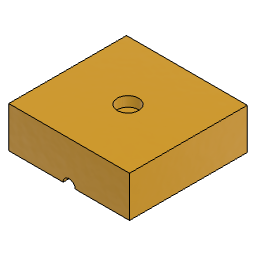
Tool change - one magnet (Autodesk Fusion 360 design; units mm, degrees)
Autodesk Fusion 360 part; units mm, degrees
note: some values were not read from the file. Chosen so that the rebuilt part matches the saved one: which face or edge a step refers to.
sketch "Sketch1" plane through (0, 0, 0) normal (0, 0, 1) x (1, 0, 0)
  line L0 (0, 1.3314) -> (42, 1.3314)
  line L1 (42, 1.3314) -> (42, 43.3314)
  line L2 (42, 43.3314) -> (0, 43.3314)
  line L3 (0, 43.3314) -> (0, 1.3314)
  dimension "d1" = 42
  dimension "d2" = 42
  constraint horizontal L0
  constraint vertical L1
  constraint horizontal L2
  constraint vertical L3
  measures "d1" distance of L0.start L2.end
  measures "d2" distance of L0.start L0.end
extrude "Extrude1" add sketch "Sketch1" along normal blind 7
sketch "Sketch2" plane through (0, 0, 7) normal (0, 0, 1) x (-1, 0, 0)
  line L0 (0, -43.3314) -> (0, -1.3314)
  line L1 (0, -1.3314) -> (-42, -1.3314)
  line L2 (-42, -1.3314) -> (-42, -43.3314)
  line L3 (-42, -43.3314) -> (0, -43.3314)
  circle A0 centre (-13, -22.3314) radius 3.55
  circle A1 centre (-29, -23.2838) radius 3.55
  dimension "d5" = 7.1
  dimension "d6" = 7.1
  dimension "d7" = 13
  dimension "d8" = 13
  dimension "d9" = 21
  measures "d5" diameter of A0
  measures "d6" diameter of A1
  measures "d7" distance of L0 A0.centre
  measures "d8" distance of L2 A1.centre
  measures "d9" distance of L1 A0.centre
sketch "Sketch4" plane through (0, 0, 7) normal (0, 0, 1) x (-1, 0, 0)
  line L0 (0, -43.3314) -> (0, -1.3314)
  line L1 (0, -1.3314) -> (-42, -1.3314)
  line L2 (-42, -1.3314) -> (-42, -43.3314)
  line L3 (-42, -43.3314) -> (0, -43.3314)
  circle A0 centre (-21, -22.3314) radius 3.55
  dimension "d12" = 7.1
  dimension "d13" = 21
  dimension "d14" = 21
  measures "d12" diameter of A0
  measures "d13" distance of L3 A0.centre
  measures "d14" distance of L0 A0.centre
extrude "Extrude3" cut sketch "Sketch4" against normal blind 3.3 contours A0
sketch "Sketch5" plane through (0, 0, 0) normal (0, 0, -1) x (1, 0, 0)
  line L0 (0, -1.3314) -> (0, -43.3314)
  line L1 (0, -43.3314) -> (42, -43.3314)
  line L2 (42, -43.3314) -> (42, -1.3314)
  line L3 (42, -1.3314) -> (0, -1.3314)
sketch "Sketch6" plane through (0, 0, 0) normal (0, 0, -1) x (1, 0, 0)
sketch "Sketch7" plane through (0, 0, 0) normal (0, 0, -1) x (1, 0, 0)
  line L0 (5.5, -6.1414) -> (36.5, -6.1414)
  line L1 (36.5, -6.1414) -> (36.5, -38.5214)
  line L2 (36.5, -38.5214) -> (5.5, -38.5214)
  line L3 (5.5, -38.5214) -> (5.5, -6.1414)
  line L4 (0, -1.3314) -> (0, -43.3314)
  line L5 (0, -43.3314) -> (42, -43.3314)
  line L6 (19, -6.1414) -> (23, -6.1414)
  line L7 (23, -6.1414) -> (23, -1)
  line L8 (23, -1) -> (19, -1)
  line L9 (19, -1) -> (19, -6.1414)
  line L10 (15.15, -38.5214) -> (26.85, -38.5214)
  line L11 (26.85, -38.5214) -> (26.85, -44)
  line L12 (26.85, -44) -> (15.15, -44)
  line L13 (15.15, -44) -> (15.15, -38.5214)
  line L14 (0, -1.3314) -> (42, -1.3314)
  line L15 (42, -1.3314) -> (42, -43.3314)
  line L16 (42, -43.3314) -> (0, -43.3314)
  line L17 (0, -43.3314) -> (0, -1.3314)
  dimension "d17" = 31
  dimension "d18" = 32.38
  dimension "d19" = 5.5
  dimension "d20" = 4.81
  dimension "d21" = 4
  dimension "d22" = 13.5
  dimension "d23" = 11.7
  dimension "d24" = 9.65
  constraint horizontal L0
  constraint vertical L1
  constraint horizontal L2
  constraint vertical L3
  constraint horizontal L6
  constraint vertical L7
  constraint horizontal L8
  constraint vertical L9
  constraint coincident L0 L6.start
  constraint horizontal L10
  constraint vertical L11
  constraint horizontal L12
  constraint vertical L13
  constraint coincident L2 L10.start
  constraint horizontal L14
  constraint vertical L15
  constraint horizontal L16
  constraint vertical L17
  constraint coincident L5.end L15.end
  constraint coincident L4.start L14.start
  measures "d17" distance of L0.start L0.end
  measures "d18" distance of L0.end L1.end
  measures "d19" distance of L3 L4
  measures "d20" distance of L2 L5
  measures "d21" distance of L7.end L8.end
  measures "d22" distance of L3 L9
  measures "d23" distance of L11.end L12.end
  measures "d24" distance of L3 L13
extrude "Extrude4" add sketch "Sketch7" along normal blind 6.55 contours L0 L2 L3 L4 L5 L9 L13 L14 L16 L17 | L0 L1 L2 L5 L7 L11 L14 L15 L16
sketch "Sketch8" plane through (0, 0, -6.55) normal (0, 0, -1) x (1, 0, 0)
  line L0 (15.15, -43.3314) -> (15.15, -38.5214)
  line L1 (15.15, -38.5214) -> (5.5, -38.5214)
  line L2 (5.5, -38.5214) -> (5.5, -6.1414)
  line L3 (5.5, -6.1414) -> (19, -6.1414)
  line L4 (19, -6.1414) -> (19, -1.3314)
  line L5 (19, -1.3314) -> (0, -1.3314)
  line L6 (0, -1.3314) -> (0, -43.3314)
  line L7 (0, -43.3314) -> (15.15, -43.3314)
sketch "Sketch9" plane through (0, 6.1414, 0) normal (0, 1, 0) x (-1, 0, 0)
  line L0 (-23, 0) -> (-36.5, 0)
  line L1 (-36.5, 0) -> (-36.5, -6.55)
  line L2 (-36.5, -6.55) -> (-23, -6.55)
  line L3 (-23, -6.55) -> (-23, 0)
sketch "Sketch10" plane through (0, 6.1414, 0) normal (0, 1, 0) x (-1, 0, 0)
  line L0 (-18.9881, 0) -> (-22.9881, 0)
  line L1 (-22.9881, 0) -> (-22.9881, -6.55)
  line L2 (-22.9881, -6.55) -> (-18.9881, -6.55)
  line L3 (-18.9881, -6.55) -> (-18.9881, 0)
  circle A0 centre (-20.9881, -6.55) radius 2
  dimension "d27" = 6.55
  dimension "d28" = 4
  dimension "d29" = 4
  constraint horizontal L0
  constraint vertical L1
  constraint horizontal L2
  constraint vertical L3
  constraint midpoint L2 A0.centre
  measures "d27" distance of L0.start L2.end
  measures "d28" distance of L1.end L2.end
  measures "d29" diameter of A0
sketch "Sketch11" plane through (0, 0, -6.55) normal (0, 0, -1) x (1, 0, 0)
  line L0 (23, -6.1414) -> (36.5, -6.1414)
  line L1 (36.5, -6.1414) -> (36.5, -38.5214)
  line L2 (36.5, -38.5214) -> (26.85, -38.5214)
  line L3 (26.85, -38.5214) -> (26.85, -43.3314)
  line L4 (26.85, -43.3314) -> (42, -43.3314)
  line L5 (42, -43.3314) -> (42, -1.3314)
  line L6 (42, -1.3314) -> (23, -1.3314)
  line L7 (23, -1.3314) -> (23, -6.1414)
sketch "Sketch12" plane through (0, 0, -6.55) normal (0, 0, -1) x (1, 0, 0)
extrude "Extrude9" add sketch "Sketch11" sketch "Sketch8" along normal blind 2 of sketch 2
sketch "Sketch22" plane through (0, 43.3314, 0) normal (0, 1, 0) x (-1, 0, 0)
  line L0 (-26.85, 0) -> (-15.15, 0)
  line L1 (-15.15, 0) -> (-15.15, -8.55)
  line L2 (-15.15, -8.55) -> (0, -8.55)
  line L3 (0, -8.55) -> (0, 7)
  line L4 (0, 7) -> (-42, 7)
  line L5 (-42, 7) -> (-42, -8.55)
  line L6 (-42, -8.55) -> (-26.85, -8.55)
  line L7 (-26.85, -8.55) -> (-26.85, 0)
  circle A0 centre (-21, -8) radius 5.85
  dimension "d42" = 11.7
  measures "d42" diameter of A0
sketch "Sketch23" plane through (0, 6.1414, 0) normal (0, 1, 0) x (-1, 0, 0)
sketch "Sketch24" plane through (0, 0, -8.55) normal (0, 0, -1) x (1, 0, 0)
  line L0 (23, -1.3314) -> (23, -6.1414)
  line L1 (23, -6.1414) -> (36.5, -6.1414)
  line L2 (36.5, -6.1414) -> (36.5, -38.5214)
  line L3 (36.5, -38.5214) -> (26.85, -38.5214)
  line L4 (26.85, -38.5214) -> (26.85, -43.3314)
  line L5 (26.85, -43.3314) -> (42, -43.3314)
  line L6 (42, -43.3314) -> (42, -1.3314)
  line L7 (42, -1.3314) -> (23, -1.3314)
sketch "Sketch25" plane through (0, 43.3314, 0) normal (0, 1, 0) x (-1, 0, 0)
extrude "Extrude10" add sketch "Sketch22" against normal blind 4.81 contours L0 L1 L7 A0
sketch "Sketch26" plane through (0, 6.1414, 0) normal (0, 1, 0) x (-1, 0, 0)
sketch "Sketch27" plane through (0, 1.3314, 0) normal (0, -1, 0) x (1, 0, 0)
  line L0 (19, 0) -> (23, 0)
  line L1 (23, 0) -> (23, -8.55)
  line L2 (23, -8.55) -> (42, -8.55)
  line L3 (42, -8.55) -> (42, 7)
  line L4 (42, 7) -> (0, 7)
  line L5 (0, 7) -> (0, -8.55)
  line L6 (0, -8.55) -> (19, -8.55)
  line L7 (19, -8.55) -> (19, 0)
  line L8 (23, -8.55) -> (19, -8.55)
  line L9 (23, -8.55) -> (23, 0)
  line L10 (19, -8.55) -> (19, 0)
  line L11 (23, 0) -> (19, 0)
  circle A0 centre (21, -8.55) radius 2
  dimension "d45" = 4
  constraint coincident L1.end L2.start
  constraint coincident L6.end L7.start
  constraint coincident L0.end L1.start
  constraint coincident L0.start L7.end
  constraint midpoint L8 A0.centre
  measures "d45" diameter of A0
extrude "Extrude11" add sketch "Sketch27" against normal blind 4.81 contours L0 L1 L7 L9 L10 L11 A0
sketch "Sketch28" plane through (36.5, 0, 0) normal (-1, 0, 0) x (0, -1, 0)
  line L0 (-6.1414, 0) -> (-38.5214, 0)
  line L1 (-38.5214, 0) -> (-38.5214, -8.55)
  line L2 (-38.5214, -8.55) -> (-6.1414, -8.55)
  line L3 (-6.1414, -8.55) -> (-6.1414, 0)
extrude "Extrude12" cut 1 faces at (0, 29.3314, -3.3667) along direction (1, 0, 0) blind 2
extrude "Extrude13" cut 1 faces at (42, 29.3314, 1.8167) along direction (-1, 0, 0) blind 2
extrude "Extrude14" cut 1 faces at (20.9502, 1.3314, 2.4815) along direction (0, 1, 0) blind 1.5
extrude "Extrude15" cut 1 faces at (6.5764, 43.3314, -2.3373) along direction (0, -1, 0) blind 1.5
sketch "Sketch29" plane through (0, 0, -8.55) normal (0, 0, -1) x (1, 0, 0)
  line L0 (2, -41.8314) -> (15.15, -41.8314)
  line L1 (15.15, -41.8314) -> (15.15, -38.5214)
  line L2 (15.15, -38.5214) -> (5.5, -38.5214)
  line L3 (5.5, -38.5214) -> (5.5, -6.1414)
  line L4 (5.5, -6.1414) -> (19, -6.1414)
  line L5 (19, -6.1414) -> (19, -2.8314)
  line L6 (19, -2.8314) -> (2, -2.8314)
  line L7 (2, -2.8314) -> (2, -41.8314)
extrude "Extrude16" add 1 faces at (20.9502, 2.8314, 2.4815) along direction (0, -1, 0) blind 0.5
extrude "Extrude17" add 1 faces at (6.5764, 41.8314, -2.3373) along direction (0, 1, 0) blind 0.5
extrude "Extrude18" add 1 faces at (40, 15.6647, 1.8167) along direction (1, 0, 0) blind 0.5
extrude "Extrude19" add 1 faces at (2, 15.6647, 1.8167) along direction (-1, 0, 0) blind 0.5
extrude "Extrude20" add 1 faces at (1.5, 15.6647, 1.8167) along direction (-1, 0, 0) blind 1
extrude "Extrude21" add 1 faces at (40.5, 15.6647, 1.8167) along direction (1, 0, 0) blind 1
sketch "Sketch30" plane through (0, 0, -8.55) normal (0, 0, -1) x (1, 0, 0)
  line L0 (41.5, -2.3314) -> (23, -2.3314)
  line L1 (23, -2.3314) -> (23, -6.1414)
  line L2 (23, -6.1414) -> (36.5, -6.1414)
  line L3 (36.5, -6.1414) -> (36.5, -38.5214)
  line L4 (36.5, -38.5214) -> (26.85, -38.5214)
  line L5 (26.85, -38.5214) -> (26.85, -42.3314)
  line L6 (26.85, -42.3314) -> (41.5, -42.3314)
  line L7 (41.5, -42.3314) -> (41.5, -2.3314)
extrude "Extrude22" cut 1 faces at (5.5764, 42.3314, -2.3373) along direction (0, -1, 0) blind 0.5
extrude "Extrude23" cut 1 faces at (21.0498, 2.3314, 2.4815) along direction (0, 1, 0) blind 0.5
extrude "Extrude24" cut 1 faces at (0.5, 15.8314, 1.8167) along direction (1, 0, 0) blind 0.5
extrude "Extrude25" cut 1 faces at (41.5, 15.8314, 1.8167) along direction (-1, 0, 0) blind 0.5
sketch "Sketch31" plane through (0, 0, -8.55) normal (0, 0, -1) x (1, 0, 0)
  line L0 (1, -2.8314) -> (1, -41.8314)
  line L1 (1, -41.8314) -> (15.15, -41.8314)
  line L2 (15.15, -41.8314) -> (15.15, -38.5214)
  line L3 (15.15, -38.5214) -> (5.5, -38.5214)
  line L4 (5.5, -38.5214) -> (5.5, -6.1414)
  line L5 (5.5, -6.1414) -> (19, -6.1414)
  line L6 (19, -6.1414) -> (19, -2.8314)
  line L7 (19, -2.8314) -> (1, -2.8314)
sketch "Sketch32" plane through (0, 0, -8.55) normal (0, 0, -1) x (1, 0, 0)
  line L0 (1, -2.8314) -> (1, -41.8314)
  line L1 (1, -41.8314) -> (15.15, -41.8314)
  line L2 (15.15, -41.8314) -> (15.15, -38.5214)
  line L3 (15.15, -38.5214) -> (5.5, -38.5214)
  line L4 (5.5, -38.5214) -> (5.5, -6.1414)
  line L5 (5.5, -6.1414) -> (19, -6.1414)
  line L6 (19, -6.1414) -> (19, -2.8314)
  line L7 (19, -2.8314) -> (1, -2.8314)
extrude "Extrude26" add 1 faces at (15.8333, 27.7281, 0) along direction (0, 0, -1) blind 2
extrude "Extrude27" cut 1 faces at (35.5167, 22.3314, 7) along direction (0, 0, -1) blind 2
extrude "Extrude28" cut 1 faces at (20.7445, 21.2299, 3.7) along direction (0, 0, -1) blind 2
extrude "Extrude5" [suppressed]
sketch "Sketch14" plane through (0, 0, -6.55) normal (0, 0, -1) x (1, 0, 0)
sketch "Sketch15" plane through (0, 43.3314, 0) normal (0, 1, 0) x (-1, 0, 0)
  line L0 (-26.85, 0) -> (-15.15, 0)
  line L1 (-15.15, 0) -> (-15.15, -6.55)
  line L2 (-15.15, -6.55) -> (0, -6.55)
  line L3 (0, -6.55) -> (0, 7)
  line L4 (0, 7) -> (-42, 7)
  line L5 (-42, 7) -> (-42, -6.55)
  line L6 (-42, -6.55) -> (-26.85, -6.55)
  line L7 (-26.85, -6.55) -> (-26.85, 0)
  line L8 (-15.15, -6.55) -> (-26.85, -6.55)
  line L9 (-26.85, -6.55) -> (-26.85, 0)
  line L10 (-26.85, 0) -> (-15.15, 0)
  line L11 (-15.15, 0) -> (-15.15, -6.55)
  circle A0 centre (-21, -6.55) radius 5.85
  dimension "d32" = 11.7
  constraint horizontal L8
  constraint vertical L9
  constraint horizontal L10
  constraint vertical L11
  constraint coincident L0.start L7.end
  constraint coincident L1.end L2.start
  constraint midpoint L8 A0.centre
  measures "d32" diameter of A0
extrude "Extrude6" [suppressed]
extrude "Extrude7" [suppressed]
sketch "Sketch16" plane through (0, 1.3314, 0) normal (0, -1, 0) x (1, 0, 0)
  line L0 (18.9881, -6.55) -> (18.9881, 0)
  line L1 (18.9881, 0) -> (23, 0)
  line L2 (23, 0) -> (23, -6.55)
  line L3 (23, -6.55) -> (42, -6.55)
  line L4 (42, -6.55) -> (42, 7)
  line L5 (42, 7) -> (0, 7)
  line L6 (0, 7) -> (0, -6.55)
  line L7 (0, -6.55) -> (18.9881, -6.55)
  line L8 (23, -6.55) -> (18.9881, -6.55)
  line L9 (18.9881, -6.55) -> (18.9881, 0)
  line L10 (18.9881, 0) -> (23, 0)
  line L11 (23, 0) -> (23, -6.55)
  circle A0 centre (20.9941, -6.55) radius 2.006
  dimension "d37" = 4.012
  constraint horizontal L8
  constraint vertical L9
  constraint horizontal L10
  constraint vertical L11
  constraint coincident L0.end L1.start
  constraint coincident L2.end L3.start
  constraint midpoint L8 A0.centre
  measures "d37" diameter of A0
extrude "Extrude8" [suppressed]
sketch "Sketch17" plane through (0, 0, 3.7) normal (0, 0, 1) x (-1, 0, 0)
  circle A0 centre (-21, -22.3314) radius 3.55
sketch "Sketch18" plane through (0, 0, 0) normal (0, 0, -1) x (1, 0, 0)
sketch "Sketch19" plane through (0, 1.3314, 0) normal (0, -1, 0) x (1, 0, 0)
  line L0 (18.9881, -6.55) -> (18.9881, -6.533)
  arc A0 (23, -6.533) -> (18.9881, -6.533) centre (20.9941, -6.55) ccw
  line L1 (23, -6.533) -> (23, -6.55)
  line L2 (23, -6.55) -> (42, -6.55)
  line L3 (42, -6.55) -> (42, 7)
  line L4 (42, 7) -> (0, 7)
  line L5 (0, 7) -> (0, -6.55)
  line L6 (0, -6.55) -> (18.9881, -6.55)
sketch "Sketch20" plane through (0, 1.3314, 0) normal (0, -1, 0) x (1, 0, 0)
sketch "Sketch21" plane through (0, 1.3314, 0) normal (0, -1, 0) x (1, 0, 0)
sketch "Sketch13" plane through (0, 0, -6.55) normal (0, 0, -1) x (1, 0, 0)
extrude "Extrude2" [suppressed]
sketch "Sketch3" plane through (0, 0, 7) normal (0, 0, 1) x (-1, 0, 0)
  circle A0 centre (-13, -22.3314) radius 3.55
  circle A1 centre (-29, -23.2838) radius 3.55
  line L0 (0, -43.3314) -> (0, -1.3314)
  line L1 (0, -1.3314) -> (-42, -1.3314)
  line L2 (-42, -1.3314) -> (-42, -43.3314)
  line L3 (-42, -43.3314) -> (0, -43.3314)
